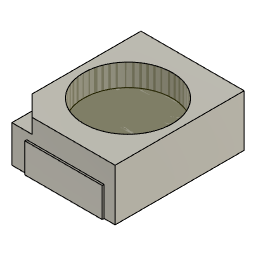
LED3528_PLCC v1 (Autodesk Fusion 360 design; units mm, degrees)
Autodesk Fusion 360 part; units mm, degrees
sketch "Sketch1" plane through (0, 0, 0) normal (0, 0, 1) x (1, 0, 0)
  line L0 (-1.4, 1.75) -> (1.4, 1.75)
  line L1 (1.4, 1.75) -> (1.4, -1.75)
  line L2 (1.4, -1.75) -> (-1.4, -1.75)
  line L3 (-1.4, -1.75) -> (-1.4, 1.75)
  circle A0 centre (0, 0) radius 1.2
  line L4 (-0.85, -1.75) -> (-1.4, -1.2)
  line L5 (-1, 1.8) -> (1.1, 1.8)
  line L6 (1.1, -1.8) -> (-1, -1.8)
  line L7 (-1, 1.75) -> (-1, 1.8)
  line L8 (1.1, 1.8) -> (1.1, 0.4796)
  line L9 (1.1, -1.75) -> (1.1, -1.8)
  line L10 (-1, -1.8) -> (-1, -1.75)
  dimension "d3" = 2.4
  constraint horizontal L0
  constraint vertical L1
  constraint horizontal L2
  constraint vertical L3
  constraint coincident A0.centre origin
  constraint coincident L2 L4.start
  constraint coincident L3 L4.end
  constraint horizontal L5
  constraint vertical L8
  constraint horizontal L6
  constraint vertical L10
  constraint coincident L0 L7.start
  constraint collinear L7 L10
  constraint coincident L2 L9.start
  constraint collinear L8 L9
  constraint coincident L2 L10.end
  constraint coincident A0 L8.end
  measures "d3" diameter of A0
extrude "Extrude1" add sketch "Sketch1" along normal blind 1.4 contours L0 L1 L2 L3 L4 makes body 1
extrude "Extrude2" add sketch "Sketch1" along normal blind 0.8 contours A0 bodies 1
extrude "Extrude3" add sketch "Sketch1" along normal blind 1 contours L2 L3 L4 bodies 1
extrude "Extrude4" add 1 faces at (-0.3517, 0.6444, 0.8) along direction (0, 0, 1) blind 0.6 separate body on bodies 1 makes body 2
extrude "Extrude5" add sketch "Sketch1" along normal blind 0.8 separate body contours L0 L5 L7 L8 | L2 L6 L9 L10 makes body 3 at (-0.3, 1.8, 0.2667) makes body 4 at (0.4, -1.75, 0.2667)
